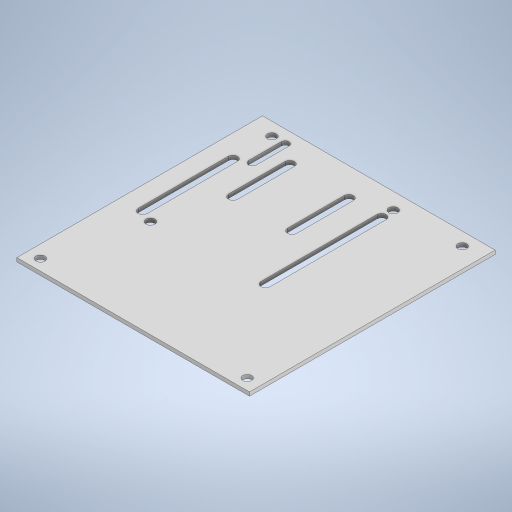
# Autodesk Inventor part: empty_board
Saved by Autodesk Inventor 2023 (Build 270158000, 158)
## iProperties
Created: 2023-03-23
Part Number: empty_board
Material: 一般
Document SubType Name: Modeling
Designer: 310611102
Density: 1 g/cm^3
Appearance: 預設
Author: 310611102
Autodesk Inventor part; units mm, degrees
ref_plane "YZ Plane" through (0, 0, 0) normal (1, 0, 0) x (0, 1, 0)
ref_plane "XZ Plane" through (0, 0, 0) normal (0, 1, 0) x (-1, 0, 0)
ref_plane "XY Plane" through (0, 0, 0) normal (0, 0, 1) x (1, 0, 0)
sketch "Sketch1" plane through (0, 0, 0) normal (0, 1, 0) x (-1, 0, 0)
  line L0 (45, 47.5) -> (-45, 47.5)
  line L1 (-45, 47.5) -> (-45, -47.5)
  line L2 (-45, -47.5) -> (45, -47.5)
  line L3 (45, -47.5) -> (45, 47.5)
  line L4 (45, 47.5) -> (-45, -47.5) construction
  line L5 (-45, 47.5) -> (45, -47.5) construction
  point P0 (0, 0)
  dimension "d0" = 95
  dimension "d1" = 90
  constraints: 12 end point, 2 midpoint, 2 parallel, 1 horizontal, 1 perpendicular
  measures "d0" distance of L2.end L0.start
  measures "d1" distance of L1.end L2.end
extrude "Extrusion1" add sketch "Sketch1" along normal blind 1.45
sketch "Sketch2" plane through (0, 1.45, 0) normal (0, 1, 0) x (1, 0, 0)
  circle A0 centre (37.38, 42.42) radius 1.75
  circle A1 centre (-40.09, -43.305) radius 1.75
  circle A2 centre (39.92, -43.305) radius 1.75
  circle A3 centre (-36.28, 42.42) radius 1.75
  line L0 (-45, 47.5) -> (-45, -47.5) projected
  line L1 (45, 47.5) -> (-45, 47.5) projected
  line L2 (45, -47.5) -> (45, 47.5) projected
  point P0 (0, 0)
  dimension "d4" = 3.5
  dimension "d5" = 3.5
  dimension "d6" = 3.5
  dimension "d7" = 3.5
  dimension "d46" = 73.66
  dimension "d47" = 7.62
  dimension "d48" = 5.08
  dimension "d49" = 85.725
  dimension "d50" = 80.01
  dimension "d51" = 2.54
  constraints: 4 centre point, 2 horizontal alignment
  measures "d4" diameter of A3
  measures "d5" diameter of A0
  measures "d6" diameter of A2
  measures "d7" diameter of A1
  measures "d46" distance of A3.centre A0.centre
  measures "d47" distance from line of L2 A0.centre
  measures "d48" distance from line of L1 A0.centre
  measures "d49" vertical distance of A2.centre A0.centre
  measures "d50" distance of A1.centre A2.centre
  measures "d51" horizontal distance of A2.centre A0.centre
extrude "Extrusion2" cut sketch "Sketch2" against normal through all
sketch "Sketch3" plane through (0, 1.45, 0) normal (0, 1, 0) x (1, 0, 0)
  circle A0 centre (-36.28, 42.42) radius 1.75
  circle A1 centre (11.98, 41.15) radius 1.75
  line L0 (45, 47.5) -> (-45, 47.5) projected
  circle A2 centre (-31.2, -9.65) radius 1.75
  circle A3 centre (-36.28, 42.42) radius 1.75 projected
  point P0 (0, 0)
  dimension "d18" = 3.5
  dimension "d19" = 3.5
  dimension "d22" = 48.26
  dimension "d23" = 1.27
  dimension "d24" = 3.5
  dimension "d25" = 5.08
  dimension "d26" = 52.07
  dimension "d44" = 0
  dimension "d45" = 0
  constraints: 3 centre point
  measures "d18" diameter of A0
  measures "d19" diameter of A1
  measures "d22" horizontal distance of A1.centre A0.centre
  measures "d23" vertical distance of A1.centre A0.centre
  measures "d24" diameter of A2
  measures "d25" horizontal distance of A0.centre A2.centre
  measures "d26" vertical distance of A0.centre A2.centre
  measures "d44" distance of A3.centre A0.centre
  measures "d45" distance of A3.centre A0.centre
extrude "Extrusion3" cut sketch "Sketch3" against normal blind 10
sketch "Sketch4" plane through (0, 1.45, 0) normal (0, 1, 0) x (1, 0, 0)
  line L0 (-36.28, 27.42) -> (-36.28, -7.58) construction
  line L1 (-38.03, 27.42) -> (-38.03, -7.58)
  line L2 (-34.53, -7.58) -> (-34.53, 27.42)
  arc A0 (-34.53, 27.42) -> (-38.03, 27.42) centre (-36.28, 27.42) ccw
  arc A1 (-38.03, -7.58) -> (-34.53, -7.58) centre (-36.28, -7.58) ccw
  line L3 (11.98, 36.65) -> (11.98, -8.35) construction
  line L4 (10.23, 36.65) -> (10.23, -8.35)
  line L5 (13.73, -8.35) -> (13.73, 36.65)
  arc A2 (13.73, 36.65) -> (10.23, 36.65) centre (11.98, 36.65) ccw
  arc A3 (10.23, -8.35) -> (13.73, -8.35) centre (11.98, -8.35) ccw
  circle A4 centre (-36.28, 42.42) radius 1.75 projected
  circle A5 centre (11.98, 41.15) radius 1.75 projected
  line L6 (-23.58, 36.67) -> (-23.58, 14.67) construction
  line L7 (-25.33, 36.67) -> (-25.33, 14.67)
  line L8 (-21.83, 14.67) -> (-21.83, 36.67)
  arc A6 (-21.83, 36.67) -> (-25.33, 36.67) centre (-23.58, 36.67) ccw
  arc A7 (-25.33, 14.67) -> (-21.83, 14.67) centre (-23.58, 14.67) ccw
  line L9 (-0.72, 36.67) -> (-0.72, 14.67) construction
  line L10 (-2.47, 36.67) -> (-2.47, 14.67)
  line L11 (1.03, 14.67) -> (1.03, 36.67)
  arc A8 (1.03, 36.67) -> (-2.47, 36.67) centre (-0.72, 36.67) ccw
  arc A9 (-2.47, 14.67) -> (1.03, 14.67) centre (-0.72, 14.67) ccw
  line L12 (-31.2, 42.5) -> (-31.2, 29.8) construction
  line L13 (-32.7, 42.5) -> (-32.7, 29.8)
  line L14 (-29.7, 29.8) -> (-29.7, 42.5)
  arc A10 (-29.7, 42.5) -> (-32.7, 42.5) centre (-31.2, 42.5) ccw
  arc A11 (-32.7, 29.8) -> (-29.7, 29.8) centre (-31.2, 29.8) ccw
  line L15 (45, 47.5) -> (-45, 47.5) projected
  line L16 (-45, 47.5) -> (-45, -47.5) projected
  point P0 (0, 0)
  point P1 (-36.28, 9.92)
  point P2 (11.98, 14.15)
  point P3 (-23.58, 25.67)
  point P4 (-0.72, 25.67)
  point P5 (-23.58, 38.42)
  point P6 (-31.2, 36.15)
  dimension "d28" = 3.5
  dimension "d29" = 3.5
  dimension "d30" = 15
  dimension "d31" = 35
  dimension "d32" = 4.5
  dimension "d33" = 45
  dimension "d34" = 12.7
  dimension "d35" = 35.56
  dimension "d36" = 3.5
  dimension "d37" = 3.5
  dimension "d38" = 22
  dimension "d41" = 4
  dimension "d52" = 3
  dimension "d53" = 5
  dimension "d54" = 12.7
  dimension "d56" = 5.08
  constraints: 40 end point, 21 point on circle, 20 tangent, 10 centre point, 7 parallel, 5 midpoint, 3 vertical, 2 coincident, 2 horizontal alignment, 2 vertical alignment
  measures "d28" distance between parallel lines of L1 L2
  measures "d29" distance between parallel lines of L5 L4
  measures "d30" distance of L0.start A4.centre
  measures "d31" distance of L0.start L0.end
  measures "d32" distance of L3.start A5.centre
  measures "d33" distance of L3.start L3.end
  measures "d34" distance from line of L6 A4.centre
  measures "d35" distance from line of A4.centre L9
  measures "d36" distance between parallel lines of L7 L8
  measures "d37" distance between parallel lines of L11 L10
  measures "d38" distance of L6.start L6.end
  measures "d41" vertical distance of A4.centre point (-23.58, 38.42)
  measures "d52" distance between parallel lines of L14 L13
  measures "d53" distance from line of L15 L12.start
  measures "d54" distance of L12.start L12.end
  measures "d56" distance from line of L12 A4.centre
extrude "Extrusion4" cut sketch "Sketch4" against normal blind 10 contours A0 L2 A1 L1 | A2 L5 A3 L4 | A6 L8 A7 L7 | A8 L11 A9 L10 | A10 L14 A11 L13
body "Solid1"
